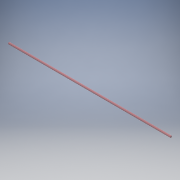
# Autodesk Inventor part: beam small 100
Saved by Autodesk Inventor 2016 (Build 200138000, 138)
## iProperties
Created: 2012-10-09
Part Number: beam small 100
Material: Laser
Document SubType Name: Modeling
Designer: cmmolo
Density: 0.001 g/cm^3
Mass: 0.0530144 g
Surface Area: 144.906 cm^2
Volume: 53.0144 cm^3
Appearance: Clear(2)
Author: cmmolo
Autodesk Inventor part; units mm, degrees
ref_plane "YZ Plane" through (0, 0, 0) normal (1, 0, 0) x (0, 1, 0)
ref_plane "XZ Plane" through (0, 0, 0) normal (0, 1, 0) x (-1, 0, 0)
ref_plane "XY Plane" through (0, 0, 0) normal (0, 0, 1) x (1, 0, 0)
sketch "Sketch2" plane through (0, 0, 0) normal (1, 0, 0) x (0, 1, 0)
  circle A0 centre (0, 0) radius 1.5
  dimension "d0" = 3
  constraints: 1 centre point, 1 coincident
  measures "d0" diameter of A0
extrude "Extrusion1" add sketch "Sketch2" along normal blind 270
body "Solid1"
